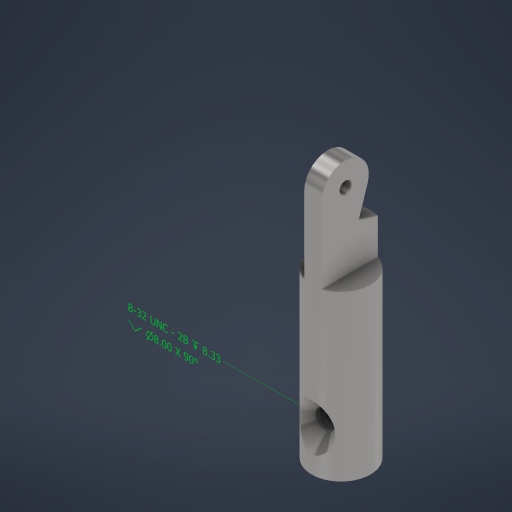
# Autodesk Inventor part: barrel_hinge-male
Saved by Autodesk Inventor 2023 (Build 270158000, 158)
## iProperties
Created: 2022-04-23
Part Number: barrel_hinge-male
Material: Stainless Steel
Document SubType Name: Modeling
Designer: Norbert Ligas
Density: 8 g/cm^3
Appearance: Semi-Polished
Author: Norbert Ligas
Autodesk Inventor part; units mm, degrees
ref_plane "XZ Plane" through (0, 0, 0) normal (0, 1, 0) x (-1, 0, 0)
sketch "Sketch1" plane through (0, 0, 0) normal (0, 1, 0) x (-1, 0, 0)
  circle A0 centre (0, 0) radius 5
  dimension "d0" = 10
  constraints: 1 centre point, 1 coincident
  measures "d0" diameter of A0
extrude "Extrusion1" add sketch "Sketch1" along normal blind 45
ref_plane "Work Plane1" through (0, 0, 5) normal (0, 0, 1) x (1, 0, 0)
sketch "Sketch2" plane through (0, 0, 5) normal (0, 0, 1) x (1, 0, 0)
  point P0 (0, 0)
  point P1 (0, 7)
  dimension "d3" = 7
  constraints: 1 vertical alignment
  measures "d3" distance of point (0, 0) point (0, 7)
hole "Hole1" at (0, 7, 5) direction (0, 0, -1) diameter 3.302 end through all countersink diameter 8 countersink angle 90 thread size "8-32 UNC" class "2B" standard "ANSI Unified Screw Threads"
sketch "Sketch5" plane through (0, 45, 0) normal (0, 1, 0) x (1, 0, 0)
  line L0 (-5, 5) -> (-1.5, 5)
  line L1 (-1.5, 5) -> (-1.5, -5)
  line L2 (-1.5, -5) -> (-5, -5)
  line L3 (-5, -5) -> (-5, 5)
  line L4 (1.5, 5) -> (5, 5)
  line L5 (5, 5) -> (5, -5)
  line L6 (5, -5) -> (1.5, -5)
  line L7 (1.5, -5) -> (1.5, 5)
  point P0 (0, 0)
  point P1 (-5, 0)
  point P2 (1.5, 0)
  point P3 (5, 0)
  point P4 (-1.5, 0)
  dimension "d16" = 3
  dimension "d17" = 10
  dimension "d18" = 10
  dimension "d27" = 5
  constraints: 16 end point, 12 horizontal alignment, 4 midpoint, 4 parallel, 2 horizontal, 2 perpendicular, 1 collinear, 1 point on line
  measures "d16" distance of L6.end L1.end
  measures "d17" distance of L5.end L2.end
  measures "d18" distance of L5.end L4.end
  measures "d27" horizontal distance of point (0, 0) L4.end
extrude "Extrusion2" cut sketch "Sketch5" against normal blind 17
sketch "Sketch6" plane through (1.5, 45, 4.7697) normal (1, 0, 0) x (0, 0, -1)
  circle A0 centre (4, -4) radius 1
  line L0 (0, 0) -> (9.5394, 0) projected
  line L1 (0, -17) -> (0, 0) projected
  point P0 (4.7697, -45)
  dimension "d32" = 2
  dimension "d33" = 4
  dimension "d34" = 4
  constraints: 1 centre point
  measures "d32" diameter of A0
  measures "d33" distance from line of L0 A0.centre
  measures "d34" distance from line of L1 A0.centre
hole "Hole2" at (1.5, 41, 0.7697) direction (-1, 0, 0) diameter 2 end through all
ref_plane "Work Plane3" through (5, 0, 0) normal (1, 0, 0) x (0, 1, 0)
sketch "Sketch10" plane through (5, 0, 0) normal (1, 0, 0) x (0, 1, 0)
  circle A0 centre (41, 0.7697) radius 4
  circle A1 centre (41, 0.7697) radius 1 projected
  line L0 (34, -5) -> (37.2338, 5)
  line L1 (28, 0.7697) -> (39.7692, -3.0362)
  line L2 (28, 4.7697) -> (28, -4.7697) projected
  line L3 (28, 4.7697) -> (45, 4.7697) projected
  line L4 (45, -5) -> (45, -4.7697) projected
  line L5 (34, -5) -> (45, -5)
  line L6 (45, 4.7697) -> (45, 5) projected
  line L7 (45, -5) -> (45, 5)
  line L8 (45, 5) -> (37.2338, 5)
  line L9 (37.2338, 5) -> (41, 4.7697)
  line L10 (45, 4.7697) -> (28, 4.7697) projected
  point P0 (0, 0)
  point P1 (45, -4.7697)
  point P2 (45, 0.7697)
  point P3 (35.1211, -1.5331)
  dimension "d54" = 8
  dimension "d55" = 6
  dimension "d56" = 4
  constraints: 12 end point, 2 horizontal, 2 point on circle, 2 point on line, 1 centre point, 1 collinear, 1 concentric, 1 perpendicular, 1 tangent
  measures "d54" diameter of A0
  measures "d55" horizontal distance of L2.end L0.start
  measures "d56" distance from line of L3 L1.start
extrude "Extrusion3" cut sketch "Sketch10" against normal through all contours L7 L4 L5 L0 L1 A0 | A0 L3 L7 | L9 L8 L6 L3
chamfer "Chamfer1" distance 2 angle 45 1 edges at (-0.2563, 8.631, -4.9934)
